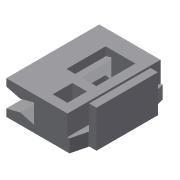
# Autodesk Inventor part: latte_d435_frame_new_legs
Saved by Autodesk Inventor 2015 (Build 190159000, 159)
## iProperties
Created: 2022-06-12
Part Number: latte_d435_frame_new_legs
Material: 常规
Document SubType Name: Modeling
Designer: chenhan
Density: 1 g/cm^3
Appearance: 默认
Author: chenhan
Autodesk Inventor part; units mm, degrees
note: some values were not read from the file. Chosen so that the rebuilt part matches the saved one: sketch regions of "拉伸3".
ref_plane "YZ Plane" through (0, 0, 0) normal (1, 0, 0) x (0, 1, 0)
ref_plane "XZ Plane" through (0, 0, 0) normal (0, 1, 0) x (-1, 0, 0)
ref_plane "XY Plane" through (0, 0, 0) normal (0, 0, 1) x (1, 0, 0)
sketch "草图1" plane through (0, 0, 0) normal (0, 1, 0) x (-1, 0, 0)
  line L0 (20, 9) -> (-20, 9)
  line L1 (-20, 9) -> (-20, -9)
  line L2 (-20, -9) -> (20, -9)
  line L3 (20, 5.1) -> (12.5, 3.2)
  line L4 (12.5, 3.2) -> (5, 5.2)
  line L5 (5, 0) -> (0, 0)
  line L6 (20, -5.1) -> (12.5, -3.2)
  line L7 (12.5, -3.2) -> (5, -5.2)
  line L8 (-13, 9) -> (-13, -9)
  line L9 (20, -9) -> (20, -5.1)
  line L10 (20, 5.1) -> (20, 9)
  line L11 (5, 5.2) -> (5, -5.2)
  line L12 (5, -5.2) -> (-20, -5.2)
  line L13 (-12.9, 9) -> (-12.9, -2)
  line L14 (-12.9, -2) -> (-16, -2)
  line L15 (-16, -2) -> (-16, 9)
  line L16 (-12.9, -2) -> (-16, -2)
  line L17 (-16, -2) -> (-16, 9)
  line L18 (-16, 9) -> (-12.9, 9)
  line L19 (-12.9, 9) -> (-12.9, -2)
  dimension "d0" = 18
  dimension "d1" = 40
  dimension "d4" = 3.9
  dimension "d6" = 5.8
  dimension "d8" = 3.8
  dimension "d13" = 33
  dimension "d14" = 11
  dimension "d15" = 3.1
  dimension "d16" = 4
  dimension "d39" = 9
  constraints: 40 end point, 6 perpendicular, 5 parallel, 5 point on line, 3 symmetric about line, 2 horizontal, 2 vertical
  measures "d0" distance of L2.end L0.start
  measures "d1" distance of L0.start L0.end
  measures "d4" distance from line of L0 L3.start
  measures "d6" distance from line of L0 L3.end
  measures "d8" distance from line of L4.end L0
  measures "d13" distance between parallel lines of L9 L8
  measures "d14" distance between parallel lines of L0 L14
  measures "d15" distance of L13.end L14.end
  measures "d16" distance between parallel lines of L1 L15
  measures "d39" distance from line of L5.start L2
extrude "拉伸1" add sketch "草图1" along normal blind 50
extrude "拉伸2" cut sketch "草图1" along normal blind 50 contours L13 L14 L8 L0 | L8 L14 L15 L0
sketch "草图2" plane through (20, 0, 9) normal (0, 0, 1) x (1, 0, 0)
  line L0 (-4, 50) -> (-4, 0) projected
  line L1 (-4, 0) -> (0, 0) projected
  line L2 (0, 0) -> (0, 50) projected
  line L3 (-4, 50) -> (0, 50) projected
  line L4 (-4, 50) -> (-4, 0) projected
  line L5 (0, 0) -> (0, 50) projected
  line L6 (-4, 8.5) -> (0, 8.5)
  line L7 (0, 8.5) -> (0, 41.5)
  line L8 (0, 41.5) -> (-4, 41.5)
  line L9 (-4, 41.5) -> (-4, 8.5)
  point P0 (-20, 0)
  point P1 (-4, 25)
  dimension "d19" = 33
  constraints: 8 end point, 2 midpoint, 2 parallel, 2 point on line, 1 horizontal, 1 perpendicular
  measures "d19" distance between parallel lines of L8 L6
extrude "拉伸3" cut sketch "草图2" against normal up to next contours L3 L2 L8 L0 | L6 L2 L1 L0
chamfer "倒角1" distance 2 distance2 8 1 edges at (16, 0, -5.5) measured on face at (6.9333, 0, 4.0667)
chamfer "倒角2" distance 2 distance2 8 1 edges at (16, 50, -5.5) measured on face at (6.9333, 50, 4.0667)
sketch "草图3" plane through (-20, 0, 9) normal (0, 0, 1) x (1, 0, 0)
  line L0 (15, 0) -> (15, 50) projected
  line L1 (15, 0) -> (15, 50) projected
  line L2 (32.9, 0) -> (32.9, 50) projected
  line L3 (11.9, 20.5) -> (27.9, 20.5)
  line L4 (27.9, 20.5) -> (27.9, 41.5)
  line L5 (27.9, 41.5) -> (11.9, 41.5)
  line L6 (11.9, 41.5) -> (11.9, 20.5)
  line L7 (0, 50) -> (32.9, 50) projected
  line L8 (20, 5) -> (27.9, 5)
  line L9 (27.9, 5) -> (27.9, 15.5)
  line L10 (27.9, 15.5) -> (20, 15.5)
  line L11 (20, 15.5) -> (20, 5)
  line L12 (0, 0) -> (32.9, 0) projected
  point P0 (20, 0)
  dimension "d28" = 21
  dimension "d29" = 8.5
  dimension "d30" = 5
  dimension "d32" = 21
  dimension "d35" = 5
  dimension "d36" = 5
  dimension "d37" = 5
  dimension "d38" = 5
  constraints: 16 end point, 4 parallel, 2 horizontal, 2 perpendicular
  measures "d28" distance of L5.end L3.start
  measures "d29" distance between parallel lines of L7 L5
  measures "d30" distance between parallel lines of L2 L4
  measures "d32" distance between parallel lines of L2 L6
  measures "d35" distance between parallel lines of L3 L10
  measures "d36" distance between parallel lines of L2 L9
  measures "d37" distance between parallel lines of L12 L8
  measures "d38" distance between parallel lines of L11 L0
extrude "拉伸4" cut sketch "草图3" against normal blind 50 contours L3 L6 L5 L0 | L0 L5 L4 L3 | L11 L10 L9 L8
sketch "草图4" plane through (-20, 0, 9) normal (0, 0, 1) x (1, 0, 0)
  line L0 (27.9, 15.5) -> (27.9, 5) projected
  line L1 (27.9, 5) -> (20, 5) projected
  line L2 (20, 5) -> (20, 15.5) projected
  line L3 (20, 15.5) -> (27.9, 15.5) projected
  line L4 (27.9, 41.5) -> (27.9, 20.5) projected
  line L5 (27.9, 20.5) -> (11.9, 20.5) projected
  line L6 (11.9, 20.5) -> (11.9, 41.5) projected
  line L7 (11.9, 41.5) -> (27.9, 41.5) projected
  line L8 (32.9, 0) -> (32.9, 50) projected
  line L9 (0, 50) -> (32.9, 50) projected
  line L10 (0, 0) -> (0, 50) projected
  line L11 (0, 0) -> (32.9, 0) projected
  line L12 (36, 8.5) -> (40, 8.5) projected
  line L13 (40, 8.5) -> (40, 41.5) projected
  line L14 (40, 41.5) -> (36, 41.5) projected
  line L15 (36, 41.5) -> (36, 8.5) projected
  point P0 (20, 0)
extrude "拉伸6" add sketch "草图4" along normal blind 2 contours L15 L14 L13 L12
